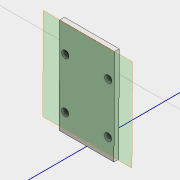
# Autodesk Inventor part: ЛЦМК000002.00.00.00.00.11
Saved by Autodesk Inventor 2021.2 (Build 252289000, 289)
## iProperties
Created: 2025-10-29
Part Number: ЛЦМК000002.00.00.00.00.11
Material: Типовые
Document SubType Name: Modeling
Designer: Захаров
Density: 1 g/cm^3
Appearance: По умолчанию
Author: Захаров
Autodesk Inventor part; units mm, degrees
ref_plane "YZ Plane" through (0, 0, 0) normal (1, 0, 0) x (0, 1, 0)
ref_plane "XZ Plane" through (0, 0, 0) normal (0, 1, 0) x (-1, 0, 0)
ref_plane "XY Plane" through (0, 0, 0) normal (0, 0, 1) x (1, 0, 0)
ref_plane "РабПлоскость1" through (0.35, 4.9821, -67.2077) normal (0, -0.006, -1) x (-1, 0, 0)
sketch "Эскиз1" plane through (0.35, 4.9821, -67.2077) normal (0, -0.006, -1) x (-1, 0, 0)
  line L0 (-11.15, 6.6878) -> (11.85, 6.6878)
  line L1 (11.85, 6.6878) -> (11.85, -33.3122)
  line L2 (11.85, -33.3122) -> (-11.15, -33.3122)
  line L3 (-11.15, -33.3122) -> (-11.15, 6.6878)
  line L4 (-11.15, 6.6878) -> (11.85, -33.3122) construction
  line L5 (11.85, 6.6878) -> (-11.15, -33.3122) construction
  point P0 (0.35, -5.3825)
  point P1 (0.35, -13.3122)
  dimension "d0" = 23
  dimension "d1" = 40
  constraints: 12 end point, 2 midpoint, 2 parallel, 1 horizontal, 1 perpendicular
  measures "d0" distance of L1.end L2.end
  measures "d1" distance of L0.end L1.end
extrude "Выдавливание1" add sketch "Эскиз1" along normal blind 2
sketch "Эскиз2" plane through (0.35, 4.9702, -69.2077) normal (0, -0.006, -1) x (-1, 0, 0)
  line L0 (-8.65, -25.5174) -> (9.35, -25.5174) construction
  line L1 (9.35, -25.5174) -> (9.35, -4.5174) construction
  line L2 (9.35, -4.5174) -> (-8.65, -4.5174) construction
  line L3 (-8.65, -4.5174) -> (-8.65, -25.5174) construction
  line L4 (-8.65, -25.5174) -> (9.35, -4.5174) construction
  line L5 (9.35, -25.5174) -> (-8.65, -4.5174) construction
  circle A0 centre (9.35, -4.5174) radius 1.5
  circle A1 centre (-8.65, -4.5174) radius 1.5
  circle A2 centre (-8.65, -25.5174) radius 1.5
  circle A3 centre (9.35, -25.5174) radius 1.5
  point P0 (0.35, -5.3825)
  point P1 (0.35, -15.0174)
  dimension "d4" = 18
  dimension "d5" = 21
  dimension "d6" = 3
  constraints: 12 end point, 4 centre point, 4 coincident, 3 equal radius, 2 midpoint, 2 parallel, 1 horizontal, 1 perpendicular
  measures "d4" distance of L2.end L1.end
  measures "d5" distance of L1.end L0.end
  measures "d6" diameter of A0
extrude "Выдавливание2" cut sketch "Эскиз2" against normal blind 2
